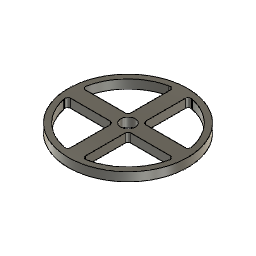
spinning_part_41mm_diameter v1 (Autodesk Fusion 360 design; units mm, degrees)
Autodesk Fusion 360 part; units mm, degrees
sketch "Sketch1" plane through (0, 0, 0) normal (0, 0, 1) x (1, 0, 0)
  circle A0 centre (0, 0) radius 20.5
  circle A1 centre (0, 0) radius 2.5
  line L0 (2.5007, 3.5) -> (2.5007, 17.1309)
  line L1 (-2.4993, 17.135) -> (-2.4993, 3.5)
  line L2 (3.5007, 2.5) -> (17.1454, 2.5)
  line L3 (17.1398, -2.5) -> (3.5007, -2.5)
  line L4 (2.5007, 0.0585) -> (2.4993, 0.0585)
  line L5 (-2.4993, -3.5) -> (-2.4993, -17.0978)
  line L6 (2.5007, -17.1125) -> (2.5007, -3.5)
  line L7 (-3.4993, 2.5) -> (-17.1847, 2.5)
  line L8 (-17.1351, -2.5) -> (-3.4993, -2.5)
  arc A2 (-3.4993, 2.5) -> (-2.4993, 3.5) centre (-3.4993, 3.5) ccw
  arc A3 (2.5007, 3.5) -> (3.5007, 2.5) centre (3.5007, 3.5) ccw
  arc A4 (3.5007, -2.5) -> (2.5007, -3.5) centre (3.5007, -3.5) ccw
  arc A5 (-2.4993, -3.5) -> (-3.4993, -2.5) centre (-3.4993, -3.5) ccw
  line L9 (3.6805, 18.1146) -> (4.1439, 18.0299)
  arc A6 (3.6805, 18.1146) -> (2.5007, 17.1309) centre (3.5007, 17.1309) ccw
  line L10 (-3.6759, 18.1193) -> (-4.0285, 18.0561)
  arc A7 (-2.4993, 17.135) -> (-3.6759, 18.1193) centre (-3.4993, 17.135) ccw
  line L11 (-18.1755, 3.6351) -> (-18.1744, 3.6434)
  arc A8 (-18.1755, 3.6351) -> (-17.1847, 2.5) centre (-17.1847, 3.5) ccw
  line L12 (-18.1194, -3.6764) -> (-18.0575, -4.0219)
  arc A9 (-17.1351, -2.5) -> (-18.1194, -3.6764) centre (-17.1351, -3.5) ccw
  line L13 (-3.7055, -18.0763) -> (-5.1082, -17.7808)
  line L14 (3.6951, -18.0935) -> (4.6802, -17.8982)
  arc A10 (-3.7055, -18.0763) -> (-2.4993, -17.0978) centre (-3.4993, -17.0978) ccw
  arc A11 (2.5007, -17.1125) -> (3.6951, -18.0935) centre (3.5007, -17.1125) ccw
  line L15 (18.1311, 3.6681) -> (18.123, 3.7158)
  line L16 (18.1248, -3.6726) -> (18.088, -3.8826)
  arc A12 (18.1248, -3.6726) -> (17.1398, -2.5) centre (17.1398, -3.5) ccw
  arc A13 (17.1454, 2.5) -> (18.1311, 3.6681) centre (17.1454, 3.5) ccw
  arc A14 (18.123, 3.7158) -> (4.1439, 18.0299) centre (0, 0) ccw
  arc A15 (4.6802, -17.8982) -> (18.088, -3.8826) centre (0, 0) ccw
  arc A16 (-4.0285, 18.0561) -> (-18.1814, 3.4188) centre (0, 0) ccw
  arc A17 (-18.0575, -4.0219) -> (-5.1082, -17.7808) centre (0, 0) ccw
  line L17 (2.4993, 0.0585) -> (2.5007, 0.0585)
  dimension "d1" = 41
  dimension "d2" = 37
  dimension "d3" = 5
  dimension "d8" = 1
  dimension "d9" = 1
  dimension "d10" = 1
  dimension "d11" = 1
  dimension "d12" = 1
  dimension "d13" = 1
  dimension "d14" = 1
  dimension "d15" = 1
  dimension "d16" = 1
  dimension "d17" = 1
  dimension "d18" = 1
  dimension "d19" = 1
  constraint coincident A0.centre A1.centre
  constraint concentric A0 A16
  constraint vertical L0
  constraint vertical L1
  constraint horizontal L2
  constraint horizontal L3
  constraint horizontal L4
  constraint vertical L5
  constraint vertical L6
  constraint horizontal L7
  constraint horizontal L8
  constraint tangent L7 A2
  constraint tangent L1 A2
  constraint coincident L4.start L0
  constraint tangent L0 A3
  constraint tangent L2 A3
  constraint coincident L4.start L6
  constraint tangent L3 A4
  constraint tangent L6 A4
  constraint tangent L8 A5
  constraint tangent L5 A5
  constraint tangent L0 A6
  constraint tangent L9 A6
  constraint tangent L10 A7
  constraint tangent L1 A7
  constraint tangent L11 A16
  constraint tangent L11 A8
  constraint tangent L7 A8
  constraint coincident L12.end A16
  constraint tangent L12 A9
  constraint tangent L8 A9
  constraint coincident L14.end A16
  constraint tangent L13 A10
  constraint tangent L5 A10
  constraint tangent L6 A11
  constraint tangent L14 A11
  constraint coincident L15.end A16
  constraint tangent L3 A12
  constraint tangent L16 A12
  constraint tangent L15 A13
  constraint tangent L2 A13
  constraint concentric A14 A16
  constraint concentric A15 A16
  constraint coincident A8 A16.end
  constraint concentric A16 A17
  constraint coincident A1 L4.end
  measures "d1" diameter of A0
  measures "d2" diameter of A16
  measures "d3" diameter of A1
  measures "d8" radius of A2
  measures "d9" radius of A3
  measures "d10" radius of A4
  measures "d11" radius of A5
  measures "d12" radius of A6
  measures "d13" radius of A7
  measures "d14" radius of A8
  measures "d15" radius of A9
  measures "d16" radius of A10
  measures "d17" radius of A11
  measures "d18" radius of A12
  measures "d19" radius of A13
extrude "Extrude1" add sketch "Sketch1" along normal blind 3
